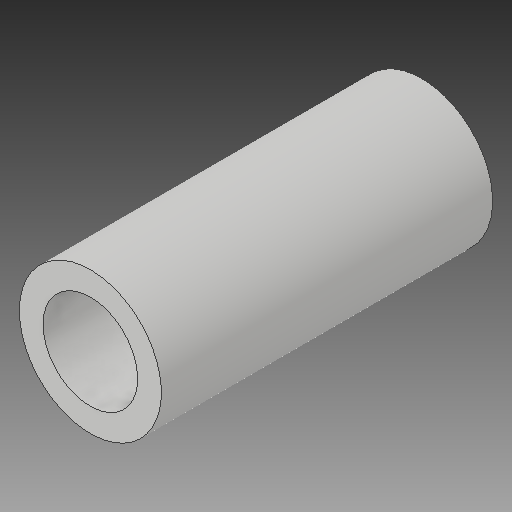
# Autodesk Inventor part: nylon_shaft_6mm
Saved by Autodesk Inventor 2017.2 (Build 212233000, 233)
## iProperties
Created: 2017-09-03
Part Number: nylon_shaft_6mm
Material: Generic
Document SubType Name: Modeling
Designer: Nic
Density: 1 g/cm^3
Appearance: Default
Author: Nic
Autodesk Inventor part; units mm, degrees
ref_plane "YZ Plane" through (0, 0, 0) normal (1, 0, 0) x (0, 1, 0)
ref_plane "XZ Plane" through (0, 0, 0) normal (0, 1, 0) x (-1, 0, 0)
ref_plane "XY Plane" through (0, 0, 0) normal (0, 0, 1) x (1, 0, 0)
sketch "Sketch1" plane through (0, 0, 0) normal (0, 1, 0) x (-1, 0, 0)
  line L0 (1, 3.5) -> (1, -3.5)
  line L1 (1, -3.5) -> (1.5, -3.5)
  line L2 (1.5, -3.5) -> (1.5, 3.5)
  line L3 (1.5, 3.5) -> (1, 3.5)
  line L4 (0, 0) -> (1.5, 0) construction
  line L5 (0, 0) -> (0, -3) construction
  dimension "d0" = 7
  dimension "d1" = 1.5
  dimension "d2" = 1
  constraints: 12 end point, 3 perpendicular, 2 vertical, 1 horizontal, 1 midpoint, 1 other
  measures "d0" distance of L1.end L2.end
  measures "d1" distance from line of L4.start L2
  measures "d2" distance from line of L4.start L0
revolve "Revolution1" add sketch "Sketch1" angle 360 about axis through (0, 0, 0) along (0, 0, -1)
body "Solid1"
